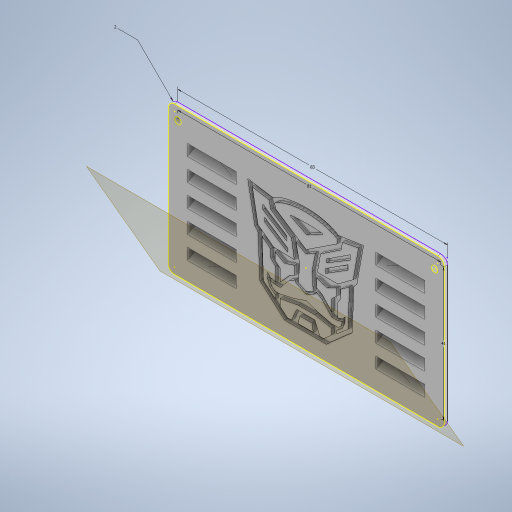
# Autodesk Inventor part: BackDoorV1
Saved by Autodesk Inventor 2024 (Build 280153000, 153)
## iProperties
Created: 2025-05-22
Part Number: BackDoorV1
Material: Ogólny
Document SubType Name: Modeling
Designer: Victoria
Density: 1 g/cm^3
Appearance: Domyślna
Author: Victoria
Autodesk Inventor part; units mm, degrees
ref_plane "YZ Plane" through (0, 0, 0) normal (1, 0, 0) x (0, 1, 0)
ref_plane "XZ Plane" through (0, 0, 0) normal (0, 1, 0) x (-1, 0, 0)
ref_plane "XY Plane" through (0, 0, 0) normal (0, 0, 1) x (1, 0, 0)
sketch "Szkic1" plane through (0, 0, 0) normal (0, 0, 1) x (1, 0, 0)
  line L0 (-40.5, -20.5) -> (40.5, -20.5)
  line L1 (40.5, -20.5) -> (40.5, 20.5)
  line L2 (40.5, 20.5) -> (-40.5, 20.5)
  line L3 (-40.5, 20.5) -> (-40.5, -20.5)
  line L4 (-40.5, -20.5) -> (40.5, 20.5) construction
  line L5 (40.5, -20.5) -> (-40.5, 20.5) construction
  line L6 (-40.5, -22) -> (40.5, -22)
  line L7 (-42.5, 20.5) -> (-42.5, -20)
  line L8 (-40.5, 23.5) -> (40.5, 23.5)
  line L9 (42.5, 21.5) -> (42.5, -20)
  line L10 (40.5, -22) -> (40.5, -22)
  line L11 (-40.5, -22) -> (-40.5, -22)
  line L12 (-42.5, 20.5) -> (-42.5, 21.5)
  line L13 (-40.5, 23.5) -> (-40.5, 23.5)
  arc A0 (-40.5, 23.5) -> (-42.5, 21.5) centre (-40.5, 21.5) ccw
  arc A1 (-42.5, -20) -> (-40.5, -22) centre (-40.5, -20) ccw
  arc A2 (40.5, -22) -> (42.5, -20) centre (40.5, -20) ccw
  arc A3 (42.5, 21.5) -> (40.5, 23.5) centre (40.5, 21.5) ccw
  point P0 (0, 0)
  point P1 (42.5, 23.5)
  point P2 (-42.5, 23.5)
  dimension "d0" = 81
  dimension "d1" = 41
  dimension "d2" = 83
  dimension "d3" = 2
  constraints: 28 end point, 8 point on circle, 8 tangent, 6 point on line, 5 perpendicular, 4 centre point, 3 equal length, 3 equal radius, 3 horizontal, 2 midpoint, 1 vertical
  measures "d0" distance of L2.end L1.end
  measures "d1" distance of L1.end L0.end
  measures "d2" distance of L8.start point (42.5, 23.5)
  measures "d3" radius of A0
extrude "Wyciągnięcie proste1" add sketch "Szkic1" along normal blind 1 contours L3 L2 L1 L0 | A1 L7 L12 A0 L8 A3 L9 A2 L6
extrude "Wyciągnięcie proste2" add sketch "Szkic1" against normal blind 2 contours L3 L2 L1 L0
sketch "Szkic2" plane through (0, 0, -2) normal (0, 0, -1) x (-1, 0, 0)
  circle A0 centre (-39.5, 19.5) radius 1
  line L0 (-40.5, -20.5) -> (-40.5, 20.5) projected
  circle A1 centre (39.5, 19.5) radius 1
  line L1 (40.5, -20.5) -> (40.5, 20.5) projected
  point P0 (0, 0)
  constraints: 2 centre point, 2 tangent
extrude "Wyciągnięcie proste3" cut sketch "Szkic2" against normal through all
sketch "Szkic3" plane through (0, 0, 1) normal (0, 0, 1) x (1, 0, 0)
  circle A0 centre (-39.5, 19.5) radius 1 projected
  circle A1 centre (39.5, 19.5) radius 1 projected
  arc A2 (-42.5, -20) -> (-40.5, -22) centre (-40.5, -20) ccw projected
  line L0 (-40.5, -22) -> (40.5, -22) projected
  arc A3 (40.5, -22) -> (42.5, -20) centre (40.5, -20) ccw projected
  line L1 (42.5, -20) -> (42.5, 21.5) projected
  arc A4 (42.5, 21.5) -> (40.5, 23.5) centre (40.5, 21.5) ccw projected
  line L2 (40.5, 23.5) -> (-40.5, 23.5) projected
  arc A5 (-40.5, 23.5) -> (-42.5, 21.5) centre (-40.5, 21.5) ccw projected
  line L3 (-42.5, 21.5) -> (-42.5, -20) projected
  line L4 (-42.5, 21.5) -> (-42.5, -20) projected
  line L5 (-16.5514, 13.3947) -> (-14.8189, 4.1445)
  line L6 (-14.8189, 4.1445) -> (-9.9927, 0.5868)
  line L7 (-9.9927, 0.5868) -> (-3.6196, 0.3702)
  line L8 (-3.6196, 0.3702) -> (-4.455, 5.7533)
  line L9 (-4.455, 5.7533) -> (-10.8899, 10.1773)
  line L10 (-10.8899, 10.1773) -> (-11.323, 12.4666)
  line L11 (-11.323, 12.4666) -> (-16.5514, 13.3947)
  line L12 (-13.303, 8.9045) -> (-13.303, 10.2966)
  line L13 (-13.303, 10.2966) -> (-5.9709, 5.6561)
  line L14 (-5.9709, 5.6561) -> (-5.9709, 4.233)
  line L15 (-5.9709, 4.233) -> (-13.303, 8.9045)
  line L16 (-12.7461, 5.8726) -> (-12.7461, 7.1101)
  line L17 (-12.7461, 7.1101) -> (-5.7234, 2.5624)
  line L18 (-5.7234, 2.5624) -> (-5.7234, 1.3558)
  line L19 (-5.7234, 1.3558) -> (-12.7461, 5.8726)
  line L20 (4.455, 5.9698) -> (10.7352, 10.1773)
  line L21 (10.7352, 10.1773) -> (11.2302, 12.4666)
  line L22 (11.2302, 12.4666) -> (16.1492, 13.3947)
  line L23 (16.1492, 13.3947) -> (14.5405, 4.1445)
  line L24 (14.5405, 4.1445) -> (9.7761, 0.5868)
  line L25 (9.7761, 0.5868) -> (3.4959, 0.5868)
  line L26 (3.4959, 0.5868) -> (4.455, 5.9698)
  line L27 (6.3421, 4.5114) -> (6.3421, 5.5633)
  line L28 (6.3421, 5.5633) -> (13.5814, 10.2966)
  line L29 (13.5814, 10.2966) -> (13.5814, 8.9045)
  line L30 (13.5814, 8.9045) -> (6.3421, 4.5114)
  line L31 (6.0018, 1.5414) -> (6.0018, 2.8408)
  line L32 (6.0018, 2.8408) -> (12.9008, 7.2957)
  line L33 (12.9008, 7.2957) -> (12.9008, 5.8726)
  line L34 (12.9008, 5.8726) -> (6.0018, 1.5414)
  line L35 (-9.4049, 11.1054) -> (-9.6833, 12.4666)
  line L36 (-9.6833, 12.4666) -> (-9.1144, 12.834)
  line L37 (-9.1144, 12.834) -> (-8.3961, 13.2106)
  line L38 (-8.3961, 13.2106) -> (-7.3824, 13.6422)
  line L39 (-7.3824, 13.6422) -> (-6.0685, 14.0739)
  line L40 (-6.0685, 14.0739) -> (-5.2975, 14.2725)
  line L41 (-5.2975, 14.2725) -> (-4.4496, 14.4505)
  line L42 (-4.4496, 14.4505) -> (-3.5244, 14.6009)
  line L43 (-3.5244, 14.6009) -> (-2.5212, 14.7168)
  line L44 (-2.5212, 14.7168) -> (-1.4394, 14.7914)
  line L45 (-1.4394, 14.7914) -> (-0.2784, 14.8179)
  line L46 (-0.2784, 14.8179) -> (0.8898, 14.7914)
  line L47 (0.8898, 14.7914) -> (1.9922, 14.7168)
  line L48 (1.9922, 14.7168) -> (3.0275, 14.6009)
  line L49 (3.0275, 14.6009) -> (3.9943, 14.4505)
  line L50 (3.9943, 14.4505) -> (4.8913, 14.2725)
  line L51 (4.8913, 14.2725) -> (5.7172, 14.0739)
  line L52 (5.7172, 14.0739) -> (7.1504, 13.6422)
  line L53 (7.1504, 13.6422) -> (8.2834, 13.2106)
  line L54 (8.2834, 13.2106) -> (9.1057, 12.834)
  line L55 (9.1057, 12.834) -> (9.7761, 12.4666)
  line L56 (9.7761, 12.4666) -> (9.4668, 11.1054)
  line L57 (9.4668, 11.1054) -> (0, 4.887)
  line L58 (0, 4.887) -> (-9.4049, 11.1054)
  line L59 (-4.8881, 11.5032) -> (0.2166, 8.9045)
  line L60 (0.2166, 8.9045) -> (5.1356, 11.5032)
  line L61 (5.1356, 11.5032) -> (5.0587, 11.5752)
  line L62 (5.0587, 11.5752) -> (4.8762, 11.6484)
  line L63 (4.8762, 11.6484) -> (4.5207, 11.7313)
  line L64 (4.5207, 11.7313) -> (3.9346, 11.8128)
  line L65 (3.9346, 11.8128) -> (3.0604, 11.8817)
  line L66 (3.0604, 11.8817) -> (1.8402, 11.9266)
  line L67 (1.8402, 11.9266) -> (0.2166, 11.9363)
  line L68 (0.2166, 11.9363) -> (-1.4151, 11.9088)
  line L69 (-1.4151, 11.9088) -> (-2.6562, 11.8556)
  line L70 (-2.6562, 11.8556) -> (-3.5603, 11.7856)
  line L71 (-3.5603, 11.7856) -> (-4.1804, 11.7081)
  line L72 (-4.1804, 11.7081) -> (-4.5699, 11.632)
  line L73 (-4.5699, 11.632) -> (-4.7822, 11.5665)
  line L74 (-4.7822, 11.5665) -> (-4.8881, 11.5032)
  line L75 (-3.0937, 5.3511) -> (0, 3.7114)
  line L76 (0, 3.7114) -> (2.8772, 5.3511)
  line L77 (2.8772, 5.3511) -> (1.8253, -0.0629)
  line L78 (1.8253, -0.0629) -> (2.2275, -5.1675)
  line L79 (2.2275, -5.1675) -> (0, -6.3432)
  line L80 (0, -6.3432) -> (-2.444, -5.1675)
  line L81 (-2.444, -5.1675) -> (-1.949, -0.0629)
  line L82 (-1.949, -0.0629) -> (-3.0937, 5.3511)
  line L83 (-7.9818, -7.7972) -> (-5.1046, -4.5488)
  line L84 (-5.1046, -4.5488) -> (-3.434, -3.6516)
  line L85 (-3.434, -3.6516) -> (-3.434, -1.022)
  line L86 (-3.434, -1.022) -> (-6.6206, -2.0738)
  line L87 (-6.6206, -2.0738) -> (-9.5596, -0.4651)
  line L88 (-9.5596, -0.4651) -> (-9.5596, -2.7854)
  line L89 (-9.5596, -2.7854) -> (-7.9818, -4.0538)
  line L90 (-7.9818, -4.0538) -> (-7.9818, -7.7972)
  line L91 (-13.5195, 1.6386) -> (-13.1483, -9.9009)
  line L92 (-13.1483, -9.9009) -> (-9.4049, -13.0565)
  line L93 (-9.4049, -13.0565) -> (-9.4049, -11.9118)
  line L94 (-9.4049, -11.9118) -> (-11.1374, -10.5197)
  line L95 (-11.1374, -10.5197) -> (-11.8489, -8.6944)
  line L96 (-11.8489, -8.6944) -> (-11.8489, -7.0857)
  line L97 (-11.8489, -7.0857) -> (-11.1374, -7.9828)
  line L98 (-11.1374, -7.9828) -> (-9.4049, -8.4778)
  line L99 (-9.4049, -8.4778) -> (-9.4049, -4.3013)
  line L100 (-9.4049, -4.3013) -> (-10.8899, -2.7854)
  line L101 (-10.8899, -2.7854) -> (-10.8899, -0.3104)
  line L102 (-10.8899, -0.3104) -> (-13.5195, 1.6386)
  line L103 (-3.434, -4.92) -> (-3.0937, -5.5035)
  line L104 (-3.0937, -5.5035) -> (-2.444, -5.7819)
  line L105 (-2.444, -5.7819) -> (0, -7.0194)
  line L106 (0, -7.0194) -> (2.3512, -5.7819)
  line L107 (2.3512, -5.7819) -> (2.8772, -5.5035)
  line L108 (2.8772, -5.5035) -> (3.2175, -4.92)
  line L109 (3.2175, -4.92) -> (4.919, -5.91)
  line L110 (4.919, -5.91) -> (7.889, -9.1584)
  line L111 (7.889, -9.1584) -> (9.7761, -9.1584)
  line L112 (9.7761, -9.1584) -> (11.2302, -8.6944)
  line L113 (11.2302, -8.6944) -> (10.7352, -10.2412)
  line L114 (10.7352, -10.2412) -> (9.7761, -10.9528)
  line L115 (9.7761, -10.9528) -> (7.889, -10.9528)
  line L116 (7.889, -10.9528) -> (3.4959, -9.9009)
  line L117 (3.4959, -9.9009) -> (0, -8.6944)
  line L118 (0, -8.6944) -> (-3.434, -9.9009)
  line L119 (-3.434, -9.9009) -> (-7.9818, -10.9528)
  line L120 (-7.9818, -10.9528) -> (-9.6833, -10.9528)
  line L121 (-9.6833, -10.9528) -> (-10.7043, -10.0512)
  line L122 (-10.7043, -10.0512) -> (-11.1374, -8.6944)
  line L123 (-11.1374, -8.6944) -> (-9.6833, -9.1584)
  line L124 (-9.6833, -9.1584) -> (-7.9818, -9.1584)
  line L125 (-7.9818, -9.1584) -> (-5.1046, -5.91)
  line L126 (-5.1046, -5.91) -> (-3.434, -4.92)
  line L127 (7.889, -13.9537) -> (5.414, -16.1502)
  line L128 (5.414, -16.1502) -> (4.2075, -16.1502)
  line L129 (4.2075, -16.1502) -> (2.6915, -12.4997)
  line L130 (2.6915, -12.4997) -> (-2.8772, -12.4997)
  line L131 (-2.8772, -12.4997) -> (-4.455, -16.1502)
  line L132 (-4.455, -16.1502) -> (-5.7234, -16.1502)
  line L133 (-5.7234, -16.1502) -> (-7.9818, -14.2631)
  line L134 (-7.9818, -14.2631) -> (-7.9818, -12.1284)
  line L135 (-7.9818, -12.1284) -> (-2.444, -11.1384)
  line L136 (-2.444, -11.1384) -> (2.6915, -11.1384)
  line L137 (2.6915, -11.1384) -> (7.889, -12.1284)
  line L138 (7.889, -12.1284) -> (7.889, -13.9537)
  line L139 (-2.444, -16.0574) -> (2.2275, -16.0574)
  line L140 (2.2275, -16.0574) -> (1.8253, -13.7681)
  line L141 (1.8253, -13.7681) -> (-1.949, -13.7681)
  line L142 (-1.949, -13.7681) -> (-2.444, -16.0574)
  line L143 (3.2175, -1.022) -> (3.2175, -3.6516)
  line L144 (3.2175, -3.6516) -> (4.919, -4.5488)
  line L145 (4.919, -4.5488) -> (7.889, -7.7972)
  line L146 (7.889, -7.7972) -> (7.889, -4.3013)
  line L147 (7.889, -4.3013) -> (9.4668, -2.7854)
  line L148 (9.4668, -2.7854) -> (9.4668, -0.6198)
  line L149 (9.4668, -0.6198) -> (6.5277, -2.0738)
  line L150 (6.5277, -2.0738) -> (3.2175, -1.022)
  line L151 (10.7352, -0.3104) -> (13.3649, 1.6386)
  line L152 (13.3649, 1.6386) -> (12.9317, -9.9009)
  line L153 (12.9317, -9.9009) -> (9.4668, -12.84)
  line L154 (9.4668, -12.84) -> (9.4668, -11.9118)
  line L155 (9.4668, -11.9118) -> (11.2302, -10.5197)
  line L156 (11.2302, -10.5197) -> (11.9727, -8.6944)
  line L157 (11.9727, -8.6944) -> (11.9727, -7.0857)
  line L158 (11.9727, -7.0857) -> (11.2302, -7.9828)
  line L159 (11.2302, -7.9828) -> (9.7761, -8.4778)
  line L160 (9.7761, -8.4778) -> (9.7761, -4.3013)
  line L161 (9.7761, -4.3013) -> (10.7352, -2.7854)
  line L162 (10.7352, -2.7854) -> (10.7352, -0.3104)
  line L163 (-6.6206, -17.2021) -> (-14.2002, -10.5197)
  line L164 (-14.2002, -10.5197) -> (-14.8189, 2.4739)
  line L165 (-14.8189, 2.4739) -> (-15.747, 3.3711)
  line L166 (-15.747, 3.3711) -> (-17.9436, 14.8179)
  line L167 (-17.9436, 14.8179) -> (-10.3021, 13.6732)
  line L168 (-10.3021, 13.6732) -> (-9.693, 14.0328)
  line L169 (-9.693, 14.0328) -> (-8.9251, 14.4041)
  line L170 (-8.9251, 14.4041) -> (-7.8426, 14.8333)
  line L171 (-7.8426, 14.8333) -> (-6.441, 15.2684)
  line L172 (-6.441, 15.2684) -> (-5.6192, 15.4718)
  line L173 (-5.6192, 15.4718) -> (-4.716, 15.657)
  line L174 (-4.716, 15.657) -> (-3.7309, 15.8176)
  line L175 (-3.7309, 15.8176) -> (-2.6633, 15.9471)
  line L176 (-2.6633, 15.9471) -> (-1.5126, 16.0388)
  line L177 (-1.5126, 16.0388) -> (-0.2784, 16.0863)
  line L178 (-0.2784, 16.0863) -> (0.9589, 16.0796)
  line L179 (0.9589, 16.0796) -> (2.1183, 16.0181)
  line L180 (2.1183, 16.0181) -> (3.1997, 15.9095)
  line L181 (3.1997, 15.9095) -> (4.2026, 15.7614)
  line L182 (4.2026, 15.7614) -> (5.1269, 15.5814)
  line L183 (5.1269, 15.5814) -> (5.9722, 15.3771)
  line L184 (5.9722, 15.3771) -> (7.4249, 14.9261)
  line L185 (7.4249, 14.9261) -> (8.5586, 14.4693)
  line L186 (8.5586, 14.4693) -> (9.3711, 14.0676)
  line L187 (9.3711, 14.0676) -> (10.0236, 13.6732)
  line L188 (10.0236, 13.6732) -> (17.6961, 14.8179)
  line L189 (17.6961, 14.8179) -> (15.6233, 3.3711)
  line L190 (15.6233, 3.3711) -> (14.757, 2.4739)
  line L191 (14.757, 2.4739) -> (14.1692, -10.2412)
  line L192 (14.1692, -10.2412) -> (6.2802, -17.2021)
  line L193 (6.2802, -17.2021) -> (-6.6206, -17.2021)
  line L194 (-14.8189, 4.1445) -> (-16.5514, 13.3947)
  line L195 (-16.5514, 13.3947) -> (-11.323, 12.4666)
  line L196 (-11.323, 12.4666) -> (-10.8899, 10.1773)
  line L197 (-10.8899, 10.1773) -> (-4.455, 5.7533)
  line L198 (-4.455, 5.7533) -> (-3.6196, 0.3702)
  line L199 (-3.6196, 0.3702) -> (-9.9927, 0.5868)
  line L200 (-9.9927, 0.5868) -> (-14.8189, 4.1445)
  line L201 (-9.6833, 12.4666) -> (-9.4049, 11.1054)
  line L202 (-9.4049, 11.1054) -> (0, 4.887)
  line L203 (0, 4.887) -> (9.4668, 11.1054)
  line L204 (9.4668, 11.1054) -> (9.7761, 12.4666)
  line L205 (9.7761, 12.4666) -> (9.1057, 12.834)
  line L206 (9.1057, 12.834) -> (8.2834, 13.2106)
  line L207 (8.2834, 13.2106) -> (7.1504, 13.6422)
  line L208 (7.1504, 13.6422) -> (5.7172, 14.0739)
  line L209 (5.7172, 14.0739) -> (4.8913, 14.2725)
  line L210 (4.8913, 14.2725) -> (3.9943, 14.4505)
  line L211 (3.9943, 14.4505) -> (3.0275, 14.6009)
  line L212 (3.0275, 14.6009) -> (1.9922, 14.7168)
  line L213 (1.9922, 14.7168) -> (0.8898, 14.7914)
  line L214 (0.8898, 14.7914) -> (-0.2784, 14.8179)
  line L215 (-0.2784, 14.8179) -> (-1.4394, 14.7914)
  line L216 (-1.4394, 14.7914) -> (-2.5212, 14.7168)
  line L217 (-2.5212, 14.7168) -> (-3.5244, 14.6009)
  line L218 (-3.5244, 14.6009) -> (-4.4496, 14.4505)
  line L219 (-4.4496, 14.4505) -> (-5.2975, 14.2725)
  line L220 (-5.2975, 14.2725) -> (-6.0685, 14.0739)
  line L221 (-6.0685, 14.0739) -> (-7.3824, 13.6422)
  line L222 (-7.3824, 13.6422) -> (-8.3961, 13.2106)
  line L223 (-8.3961, 13.2106) -> (-9.1144, 12.834)
  line L224 (-9.1144, 12.834) -> (-9.6833, 12.4666)
  line L225 (0, 3.7114) -> (-3.0937, 5.3511)
  line L226 (-3.0937, 5.3511) -> (-1.949, -0.0629)
  line L227 (-1.949, -0.0629) -> (-2.444, -5.1675)
  line L228 (-2.444, -5.1675) -> (0, -6.3432)
  line L229 (0, -6.3432) -> (2.2275, -5.1675)
  line L230 (2.2275, -5.1675) -> (1.8253, -0.0629)
  line L231 (1.8253, -0.0629) -> (2.8772, 5.3511)
  line L232 (2.8772, 5.3511) -> (0, 3.7114)
  line L233 (10.7352, 10.1773) -> (4.455, 5.9698)
  line L234 (4.455, 5.9698) -> (3.4959, 0.5868)
  line L235 (3.4959, 0.5868) -> (9.7761, 0.5868)
  line L236 (9.7761, 0.5868) -> (14.5405, 4.1445)
  line L237 (14.5405, 4.1445) -> (16.1492, 13.3947)
  line L238 (16.1492, 13.3947) -> (11.2302, 12.4666)
  line L239 (11.2302, 12.4666) -> (10.7352, 10.1773)
  line L240 (-2.444, -5.7819) -> (-3.0937, -5.5035)
  line L241 (-3.0937, -5.5035) -> (-3.434, -4.92)
  line L242 (-3.434, -4.92) -> (-5.1046, -5.91)
  line L243 (-5.1046, -5.91) -> (-7.9818, -9.1584)
  line L244 (-7.9818, -9.1584) -> (-9.6833, -9.1584)
  line L245 (-9.6833, -9.1584) -> (-11.1374, -8.6944)
  line L246 (-11.1374, -8.6944) -> (-10.7043, -10.0512)
  line L247 (-10.7043, -10.0512) -> (-9.6833, -10.9528)
  line L248 (-9.6833, -10.9528) -> (-7.9818, -10.9528)
  line L249 (-7.9818, -10.9528) -> (-3.434, -9.9009)
  line L250 (-3.434, -9.9009) -> (0, -8.6944)
  line L251 (0, -8.6944) -> (3.4959, -9.9009)
  line L252 (3.4959, -9.9009) -> (7.889, -10.9528)
  line L253 (7.889, -10.9528) -> (9.7761, -10.9528)
  line L254 (9.7761, -10.9528) -> (10.7352, -10.2412)
  line L255 (10.7352, -10.2412) -> (11.2302, -8.6944)
  line L256 (11.2302, -8.6944) -> (9.7761, -9.1584)
  line L257 (9.7761, -9.1584) -> (7.889, -9.1584)
  line L258 (7.889, -9.1584) -> (4.919, -5.91)
  line L259 (4.919, -5.91) -> (3.2175, -4.92)
  line L260 (3.2175, -4.92) -> (2.8772, -5.5035)
  line L261 (2.8772, -5.5035) -> (2.3512, -5.7819)
  line L262 (2.3512, -5.7819) -> (0, -7.0194)
  line L263 (0, -7.0194) -> (-2.444, -5.7819)
  line L264 (-13.1483, -9.9009) -> (-13.5195, 1.6386)
  line L265 (-13.5195, 1.6386) -> (-10.8899, -0.3104)
  line L266 (-10.8899, -0.3104) -> (-10.8899, -2.7854)
  line L267 (-10.8899, -2.7854) -> (-9.4049, -4.3013)
  line L268 (-9.4049, -4.3013) -> (-9.4049, -8.4778)
  line L269 (-9.4049, -8.4778) -> (-11.1374, -7.9828)
  line L270 (-11.1374, -7.9828) -> (-11.8489, -7.0857)
  line L271 (-11.8489, -7.0857) -> (-11.8489, -8.6944)
  line L272 (-11.8489, -8.6944) -> (-11.1374, -10.5197)
  line L273 (-11.1374, -10.5197) -> (-9.4049, -11.9118)
  line L274 (-9.4049, -11.9118) -> (-9.4049, -13.0565)
  line L275 (-9.4049, -13.0565) -> (-13.1483, -9.9009)
  line L276 (2.2275, -16.0574) -> (-2.444, -16.0574)
  line L277 (-2.444, -16.0574) -> (-1.949, -13.7681)
  line L278 (-1.949, -13.7681) -> (1.8253, -13.7681)
  line L279 (1.8253, -13.7681) -> (2.2275, -16.0574)
  line L280 (3.2175, -3.6516) -> (3.2175, -1.022)
  line L281 (3.2175, -1.022) -> (6.5277, -2.0738)
  line L282 (6.5277, -2.0738) -> (9.4668, -0.6198)
  line L283 (9.4668, -0.6198) -> (9.4668, -2.7854)
  line L284 (9.4668, -2.7854) -> (7.889, -4.3013)
  line L285 (7.889, -4.3013) -> (7.889, -7.7972)
  line L286 (7.889, -7.7972) -> (4.919, -4.5488)
  line L287 (4.919, -4.5488) -> (3.2175, -3.6516)
  line L288 (13.3649, 1.6386) -> (10.7352, -0.3104)
  line L289 (10.7352, -0.3104) -> (10.7352, -2.7854)
  line L290 (10.7352, -2.7854) -> (9.7761, -4.3013)
  line L291 (9.7761, -4.3013) -> (9.7761, -8.4778)
  line L292 (9.7761, -8.4778) -> (11.2302, -7.9828)
  line L293 (11.2302, -7.9828) -> (11.9727, -7.0857)
  line L294 (11.9727, -7.0857) -> (11.9727, -8.6944)
  line L295 (11.9727, -8.6944) -> (11.2302, -10.5197)
  line L296 (11.2302, -10.5197) -> (9.4668, -11.9118)
  line L297 (9.4668, -11.9118) -> (9.4668, -12.84)
  line L298 (9.4668, -12.84) -> (12.9317, -9.9009)
  line L299 (12.9317, -9.9009) -> (13.3649, 1.6386)
  line L300 (5.414, -16.1502) -> (7.889, -13.9537)
  line L301 (7.889, -13.9537) -> (7.889, -12.1284)
  line L302 (7.889, -12.1284) -> (2.6915, -11.1384)
  line L303 (2.6915, -11.1384) -> (-2.444, -11.1384)
  line L304 (-2.444, -11.1384) -> (-7.9818, -12.1284)
  line L305 (-7.9818, -12.1284) -> (-7.9818, -14.2631)
  line L306 (-7.9818, -14.2631) -> (-5.7234, -16.1502)
  line L307 (-5.7234, -16.1502) -> (-4.455, -16.1502)
  line L308 (-4.455, -16.1502) -> (-2.8772, -12.4997)
  line L309 (-2.8772, -12.4997) -> (2.6915, -12.4997)
  line L310 (2.6915, -12.4997) -> (4.2075, -16.1502)
  line L311 (4.2075, -16.1502) -> (5.414, -16.1502)
  line L312 (-5.1046, -4.5488) -> (-7.9818, -7.7972)
  line L313 (-7.9818, -7.7972) -> (-7.9818, -4.0538)
  line L314 (-7.9818, -4.0538) -> (-9.5596, -2.7854)
  line L315 (-9.5596, -2.7854) -> (-9.5596, -0.4651)
  line L316 (-9.5596, -0.4651) -> (-6.6206, -2.0738)
  line L317 (-6.6206, -2.0738) -> (-3.434, -1.022)
  line L318 (-3.434, -1.022) -> (-3.434, -3.6516)
  line L319 (-3.434, -3.6516) -> (-5.1046, -4.5488)
  line L320 (6.0018, 2.8408) -> (6.0018, 1.5414)
  line L321 (6.0018, 1.5414) -> (12.9008, 5.8726)
  line L322 (12.9008, 5.8726) -> (12.9008, 7.2957)
  line L323 (12.9008, 7.2957) -> (6.0018, 2.8408)
  line L324 (6.3421, 5.5633) -> (6.3421, 4.5114)
  line L325 (6.3421, 4.5114) -> (13.5814, 8.9045)
  line L326 (13.5814, 8.9045) -> (13.5814, 10.2966)
  line L327 (13.5814, 10.2966) -> (6.3421, 5.5633)
  line L328 (0.2166, 8.9045) -> (-4.8881, 11.5032)
  line L329 (-4.8881, 11.5032) -> (-4.7822, 11.5665)
  line L330 (-4.7822, 11.5665) -> (-4.5699, 11.632)
  line L331 (-4.5699, 11.632) -> (-4.1804, 11.7081)
  line L332 (-4.1804, 11.7081) -> (-3.5603, 11.7856)
  line L333 (-3.5603, 11.7856) -> (-2.6562, 11.8556)
  line L334 (-2.6562, 11.8556) -> (-1.4151, 11.9088)
  line L335 (-1.4151, 11.9088) -> (0.2166, 11.9363)
  line L336 (0.2166, 11.9363) -> (1.8402, 11.9266)
  line L337 (1.8402, 11.9266) -> (3.0604, 11.8817)
  line L338 (3.0604, 11.8817) -> (3.9346, 11.8128)
  line L339 (3.9346, 11.8128) -> (4.5207, 11.7313)
  line L340 (4.5207, 11.7313) -> (4.8762, 11.6484)
  line L341 (4.8762, 11.6484) -> (5.0587, 11.5752)
  line L342 (5.0587, 11.5752) -> (5.1356, 11.5032)
  line L343 (5.1356, 11.5032) -> (0.2166, 8.9045)
  line L344 (-13.303, 10.2966) -> (-13.303, 8.9045)
  line L345 (-13.303, 8.9045) -> (-5.9709, 4.233)
  line L346 (-5.9709, 4.233) -> (-5.9709, 5.6561)
  line L347 (-5.9709, 5.6561) -> (-13.303, 10.2966)
  line L348 (-12.7461, 7.1101) -> (-12.7461, 5.8726)
  line L349 (-12.7461, 5.8726) -> (-5.7234, 1.3558)
  line L350 (-5.7234, 1.3558) -> (-5.7234, 2.5624)
  line L351 (-5.7234, 2.5624) -> (-12.7461, 7.1101)
  line L352 (-16.5514, 13.3947) -> (-14.8189, 4.1445)
  line L353 (-14.8189, 4.1445) -> (-9.9927, 0.5868)
  line L354 (-9.9927, 0.5868) -> (-3.6196, 0.3702)
  line L355 (-3.6196, 0.3702) -> (-4.455, 5.7533)
  line L356 (-4.455, 5.7533) -> (-10.8899, 10.1773)
  line L357 (-10.8899, 10.1773) -> (-11.323, 12.4666)
  line L358 (-11.323, 12.4666) -> (-16.5514, 13.3947)
  line L359 (-13.303, 8.9045) -> (-13.303, 10.2966)
  line L360 (-13.303, 10.2966) -> (-5.9709, 5.6561)
  line L361 (-5.9709, 5.6561) -> (-5.9709, 4.233)
  line L362 (-5.9709, 4.233) -> (-13.303, 8.9045)
  line L363 (-12.7461, 5.8726) -> (-12.7461, 7.1101)
  line L364 (-12.7461, 7.1101) -> (-5.7234, 2.5624)
  line L365 (-5.7234, 2.5624) -> (-5.7234, 1.3558)
  line L366 (-5.7234, 1.3558) -> (-12.7461, 5.8726)
  line L367 (4.455, 5.9698) -> (10.7352, 10.1773)
  line L368 (10.7352, 10.1773) -> (11.2302, 12.4666)
  line L369 (11.2302, 12.4666) -> (16.1492, 13.3947)
  line L370 (16.1492, 13.3947) -> (14.5405, 4.1445)
  line L371 (14.5405, 4.1445) -> (9.7761, 0.5868)
  line L372 (9.7761, 0.5868) -> (3.4959, 0.5868)
  line L373 (3.4959, 0.5868) -> (4.455, 5.9698)
  line L374 (6.3421, 4.5114) -> (6.3421, 5.5633)
  line L375 (6.3421, 5.5633) -> (13.5814, 10.2966)
  line L376 (13.5814, 10.2966) -> (13.5814, 8.9045)
  line L377 (13.5814, 8.9045) -> (6.3421, 4.5114)
  line L378 (6.0018, 1.5414) -> (6.0018, 2.8408)
  line L379 (6.0018, 2.8408) -> (12.9008, 7.2957)
  line L380 (12.9008, 7.2957) -> (12.9008, 5.8726)
  line L381 (12.9008, 5.8726) -> (6.0018, 1.5414)
  line L382 (-9.4049, 11.1054) -> (-9.6833, 12.4666)
  line L383 (-9.6833, 12.4666) -> (-9.1144, 12.834)
  line L384 (-9.1144, 12.834) -> (-8.3961, 13.2106)
  line L385 (-8.3961, 13.2106) -> (-7.3824, 13.6422)
  line L386 (-7.3824, 13.6422) -> (-6.0685, 14.0739)
  line L387 (-6.0685, 14.0739) -> (-5.2975, 14.2725)
  line L388 (-5.2975, 14.2725) -> (-4.4496, 14.4505)
  line L389 (-4.4496, 14.4505) -> (-3.5244, 14.6009)
  line L390 (-3.5244, 14.6009) -> (-2.5212, 14.7168)
  line L391 (-2.5212, 14.7168) -> (-1.4394, 14.7914)
  line L392 (-1.4394, 14.7914) -> (-0.2784, 14.8179)
  line L393 (-0.2784, 14.8179) -> (0.8898, 14.7914)
  line L394 (0.8898, 14.7914) -> (1.9922, 14.7168)
  line L395 (1.9922, 14.7168) -> (3.0275, 14.6009)
  line L396 (3.0275, 14.6009) -> (3.9943, 14.4505)
  line L397 (3.9943, 14.4505) -> (4.8913, 14.2725)
  line L398 (4.8913, 14.2725) -> (5.7172, 14.0739)
  line L399 (5.7172, 14.0739) -> (7.1504, 13.6422)
  line L400 (7.1504, 13.6422) -> (8.2834, 13.2106)
  line L401 (8.2834, 13.2106) -> (9.1057, 12.834)
  line L402 (9.1057, 12.834) -> (9.7761, 12.4666)
  line L403 (9.7761, 12.4666) -> (9.4668, 11.1054)
  line L404 (9.4668, 11.1054) -> (0, 4.887)
  line L405 (0, 4.887) -> (-9.4049, 11.1054)
  line L406 (-4.8881, 11.5032) -> (0.2166, 8.9045)
  line L407 (0.2166, 8.9045) -> (5.1356, 11.5032)
  line L408 (5.1356, 11.5032) -> (5.0587, 11.5752)
  line L409 (5.0587, 11.5752) -> (4.8762, 11.6484)
  line L410 (4.8762, 11.6484) -> (4.5207, 11.7313)
  line L411 (4.5207, 11.7313) -> (3.9346, 11.8128)
  line L412 (3.9346, 11.8128) -> (3.0604, 11.8817)
  line L413 (3.0604, 11.8817) -> (1.8402, 11.9266)
  line L414 (1.8402, 11.9266) -> (0.2166, 11.9363)
  line L415 (0.2166, 11.9363) -> (-1.4151, 11.9088)
  line L416 (-1.4151, 11.9088) -> (-2.6562, 11.8556)
  line L417 (-2.6562, 11.8556) -> (-3.5603, 11.7856)
  line L418 (-3.5603, 11.7856) -> (-4.1804, 11.7081)
  line L419 (-4.1804, 11.7081) -> (-4.5699, 11.632)
  line L420 (-4.5699, 11.632) -> (-4.7822, 11.5665)
  line L421 (-4.7822, 11.5665) -> (-4.8881, 11.5032)
  line L422 (-3.0937, 5.3511) -> (0, 3.7114)
  line L423 (0, 3.7114) -> (2.8772, 5.3511)
  line L424 (2.8772, 5.3511) -> (1.8253, -0.0629)
  line L425 (1.8253, -0.0629) -> (2.2275, -5.1675)
  line L426 (2.2275, -5.1675) -> (0, -6.3432)
  line L427 (0, -6.3432) -> (-2.444, -5.1675)
  line L428 (-2.444, -5.1675) -> (-1.949, -0.0629)
  line L429 (-1.949, -0.0629) -> (-3.0937, 5.3511)
  line L430 (-7.9818, -7.7972) -> (-5.1046, -4.5488)
  line L431 (-5.1046, -4.5488) -> (-3.434, -3.6516)
  line L432 (-3.434, -3.6516) -> (-3.434, -1.022)
  line L433 (-3.434, -1.022) -> (-6.6206, -2.0738)
  line L434 (-6.6206, -2.0738) -> (-9.5596, -0.4651)
  line L435 (-9.5596, -0.4651) -> (-9.5596, -2.7854)
  line L436 (-9.5596, -2.7854) -> (-7.9818, -4.0538)
  line L437 (-7.9818, -4.0538) -> (-7.9818, -7.7972)
  line L438 (-13.5195, 1.6386) -> (-13.1483, -9.9009)
  line L439 (-13.1483, -9.9009) -> (-9.4049, -13.0565)
  line L440 (-9.4049, -13.0565) -> (-9.4049, -11.9118)
  line L441 (-9.4049, -11.9118) -> (-11.1374, -10.5197)
  line L442 (-11.1374, -10.5197) -> (-11.8489, -8.6944)
  line L443 (-11.8489, -8.6944) -> (-11.8489, -7.0857)
  line L444 (-11.8489, -7.0857) -> (-11.1374, -7.9828)
  line L445 (-11.1374, -7.9828) -> (-9.4049, -8.4778)
  line L446 (-9.4049, -8.4778) -> (-9.4049, -4.3013)
  line L447 (-9.4049, -4.3013) -> (-10.8899, -2.7854)
  line L448 (-10.8899, -2.7854) -> (-10.8899, -0.3104)
  line L449 (-10.8899, -0.3104) -> (-13.5195, 1.6386)
  line L450 (-3.434, -4.92) -> (-3.0937, -5.5035)
  line L451 (-3.0937, -5.5035) -> (-2.444, -5.7819)
  line L452 (-2.444, -5.7819) -> (0, -7.0194)
  line L453 (0, -7.0194) -> (2.3512, -5.7819)
  line L454 (2.3512, -5.7819) -> (2.8772, -5.5035)
  line L455 (2.8772, -5.5035) -> (3.2175, -4.92)
  line L456 (3.2175, -4.92) -> (4.919, -5.91)
  line L457 (4.919, -5.91) -> (7.889, -9.1584)
  line L458 (7.889, -9.1584) -> (9.7761, -9.1584)
  line L459 (9.7761, -9.1584) -> (11.2302, -8.6944)
  line L460 (11.2302, -8.6944) -> (10.7352, -10.2412)
  line L461 (10.7352, -10.2412) -> (9.7761, -10.9528)
  line L462 (9.7761, -10.9528) -> (7.889, -10.9528)
  line L463 (7.889, -10.9528) -> (3.4959, -9.9009)
  line L464 (3.4959, -9.9009) -> (0, -8.6944)
  line L465 (0, -8.6944) -> (-3.434, -9.9009)
  line L466 (-3.434, -9.9009) -> (-7.9818, -10.9528)
  line L467 (-7.9818, -10.9528) -> (-9.6833, -10.9528)
  line L468 (-9.6833, -10.9528) -> (-10.7043, -10.0512)
  line L469 (-10.7043, -10.0512) -> (-11.1374, -8.6944)
  line L470 (-11.1374, -8.6944) -> (-9.6833, -9.1584)
  line L471 (-9.6833, -9.1584) -> (-7.9818, -9.1584)
  line L472 (-7.9818, -9.1584) -> (-5.1046, -5.91)
  line L473 (-5.1046, -5.91) -> (-3.434, -4.92)
  line L474 (7.889, -13.9537) -> (5.414, -16.1502)
  line L475 (5.414, -16.1502) -> (4.2075, -16.1502)
  line L476 (4.2075, -16.1502) -> (2.6915, -12.4997)
  line L477 (2.6915, -12.4997) -> (-2.8772, -12.4997)
  line L478 (-2.8772, -12.4997) -> (-4.455, -16.1502)
  line L479 (-4.455, -16.1502) -> (-5.7234, -16.1502)
  line L480 (-5.7234, -16.1502) -> (-7.9818, -14.2631)
  line L481 (-7.9818, -14.2631) -> (-7.9818, -12.1284)
  line L482 (-7.9818, -12.1284) -> (-2.444, -11.1384)
  line L483 (-2.444, -11.1384) -> (2.6915, -11.1384)
  line L484 (2.6915, -11.1384) -> (7.889, -12.1284)
  line L485 (7.889, -12.1284) -> (7.889, -13.9537)
  line L486 (-2.444, -16.0574) -> (2.2275, -16.0574)
  line L487 (2.2275, -16.0574) -> (1.8253, -13.7681)
  line L488 (1.8253, -13.7681) -> (-1.949, -13.7681)
  line L489 (-1.949, -13.7681) -> (-2.444, -16.0574)
  line L490 (3.2175, -1.022) -> (3.2175, -3.6516)
  line L491 (3.2175, -3.6516) -> (4.919, -4.5488)
  line L492 (4.919, -4.5488) -> (7.889, -7.7972)
  line L493 (7.889, -7.7972) -> (7.889, -4.3013)
  line L494 (7.889, -4.3013) -> (9.4668, -2.7854)
  line L495 (9.4668, -2.7854) -> (9.4668, -0.6198)
  line L496 (9.4668, -0.6198) -> (6.5277, -2.0738)
  line L497 (6.5277, -2.0738) -> (3.2175, -1.022)
  line L498 (10.7352, -0.3104) -> (13.3649, 1.6386)
  line L499 (13.3649, 1.6386) -> (12.9317, -9.9009)
  line L500 (12.9317, -9.9009) -> (9.4668, -12.84)
  line L501 (9.4668, -12.84) -> (9.4668, -11.9118)
  line L502 (9.4668, -11.9118) -> (11.2302, -10.5197)
  line L503 (11.2302, -10.5197) -> (11.9727, -8.6944)
  line L504 (11.9727, -8.6944) -> (11.9727, -7.0857)
  line L505 (11.9727, -7.0857) -> (11.2302, -7.9828)
  line L506 (11.2302, -7.9828) -> (9.7761, -8.4778)
  line L507 (9.7761, -8.4778) -> (9.7761, -4.3013)
  line L508 (9.7761, -4.3013) -> (10.7352, -2.7854)
  line L509 (10.7352, -2.7854) -> (10.7352, -0.3104)
  line L510 (-6.6206, -17.2021) -> (-14.2002, -10.5197)
  line L511 (-14.2002, -10.5197) -> (-14.8189, 2.4739)
  line L512 (-14.8189, 2.4739) -> (-15.747, 3.3711)
  line L513 (-15.747, 3.3711) -> (-17.9436, 14.8179)
  line L514 (-17.9436, 14.8179) -> (-10.3021, 13.6732)
  line L515 (-10.3021, 13.6732) -> (-9.693, 14.0328)
  line L516 (-9.693, 14.0328) -> (-8.9251, 14.4041)
  line L517 (-8.9251, 14.4041) -> (-7.8426, 14.8333)
  line L518 (-7.8426, 14.8333) -> (-6.441, 15.2684)
  line L519 (-6.441, 15.2684) -> (-5.6192, 15.4718)
  line L520 (-5.6192, 15.4718) -> (-4.716, 15.657)
  line L521 (-4.716, 15.657) -> (-3.7309, 15.8176)
  line L522 (-3.7309, 15.8176) -> (-2.6633, 15.9471)
  line L523 (-2.6633, 15.9471) -> (-1.5126, 16.0388)
  line L524 (-1.5126, 16.0388) -> (-0.2784, 16.0863)
  line L525 (-0.2784, 16.0863) -> (0.9589, 16.0796)
  line L526 (0.9589, 16.0796) -> (2.1183, 16.0181)
  line L527 (2.1183, 16.0181) -> (3.1997, 15.9095)
  line L528 (3.1997, 15.9095) -> (4.2026, 15.7614)
  line L529 (4.2026, 15.7614) -> (5.1269, 15.5814)
  line L530 (5.1269, 15.5814) -> (5.9722, 15.3771)
  line L531 (5.9722, 15.3771) -> (7.4249, 14.9261)
  line L532 (7.4249, 14.9261) -> (8.5586, 14.4693)
  line L533 (8.5586, 14.4693) -> (9.3711, 14.0676)
  line L534 (9.3711, 14.0676) -> (10.0236, 13.6732)
  line L535 (10.0236, 13.6732) -> (17.6961, 14.8179)
  line L536 (17.6961, 14.8179) -> (15.6233, 3.3711)
  line L537 (15.6233, 3.3711) -> (14.757, 2.4739)
  line L538 (14.757, 2.4739) -> (14.1692, -10.2412)
  line L539 (14.1692, -10.2412) -> (6.2802, -17.2021)
  line L540 (6.2802, -17.2021) -> (-6.6206, -17.2021)
  line L541 (-14.8189, 4.1445) -> (-16.5514, 13.3947)
  line L542 (-16.5514, 13.3947) -> (-11.323, 12.4666)
  line L543 (-11.323, 12.4666) -> (-10.8899, 10.1773)
  line L544 (-10.8899, 10.1773) -> (-4.455, 5.7533)
  line L545 (-4.455, 5.7533) -> (-3.6196, 0.3702)
  line L546 (-3.6196, 0.3702) -> (-9.9927, 0.5868)
  line L547 (-9.9927, 0.5868) -> (-14.8189, 4.1445)
  line L548 (-9.6833, 12.4666) -> (-9.4049, 11.1054)
  line L549 (-9.4049, 11.1054) -> (0, 4.887)
  line L550 (0, 4.887) -> (9.4668, 11.1054)
  line L551 (9.4668, 11.1054) -> (9.7761, 12.4666)
  line L552 (9.7761, 12.4666) -> (9.1057, 12.834)
  line L553 (9.1057, 12.834) -> (8.2834, 13.2106)
  line L554 (8.2834, 13.2106) -> (7.1504, 13.6422)
  line L555 (7.1504, 13.6422) -> (5.7172, 14.0739)
  line L556 (5.7172, 14.0739) -> (4.8913, 14.2725)
  line L557 (4.8913, 14.2725) -> (3.9943, 14.4505)
  line L558 (3.9943, 14.4505) -> (3.0275, 14.6009)
  line L559 (3.0275, 14.6009) -> (1.9922, 14.7168)
  line L560 (1.9922, 14.7168) -> (0.8898, 14.7914)
  line L561 (0.8898, 14.7914) -> (-0.2784, 14.8179)
  line L562 (-0.2784, 14.8179) -> (-1.4394, 14.7914)
  line L563 (-1.4394, 14.7914) -> (-2.5212, 14.7168)
  line L564 (-2.5212, 14.7168) -> (-3.5244, 14.6009)
  line L565 (-3.5244, 14.6009) -> (-4.4496, 14.4505)
  line L566 (-4.4496, 14.4505) -> (-5.2975, 14.2725)
  line L567 (-5.2975, 14.2725) -> (-6.0685, 14.0739)
  line L568 (-6.0685, 14.0739) -> (-7.3824, 13.6422)
  line L569 (-7.3824, 13.6422) -> (-8.3961, 13.2106)
  line L570 (-8.3961, 13.2106) -> (-9.1144, 12.834)
  line L571 (-9.1144, 12.834) -> (-9.6833, 12.4666)
  line L572 (0, 3.7114) -> (-3.0937, 5.3511)
  line L573 (-3.0937, 5.3511) -> (-1.949, -0.0629)
  line L574 (-1.949, -0.0629) -> (-2.444, -5.1675)
  line L575 (-2.444, -5.1675) -> (0, -6.3432)
  line L576 (0, -6.3432) -> (2.2275, -5.1675)
  line L577 (2.2275, -5.1675) -> (1.8253, -0.0629)
  line L578 (1.8253, -0.0629) -> (2.8772, 5.3511)
  line L579 (2.8772, 5.3511) -> (0, 3.7114)
  line L580 (10.7352, 10.1773) -> (4.455, 5.9698)
  line L581 (4.455, 5.9698) -> (3.4959, 0.5868)
  line L582 (3.4959, 0.5868) -> (9.7761, 0.5868)
  line L583 (9.7761, 0.5868) -> (14.5405, 4.1445)
  line L584 (14.5405, 4.1445) -> (16.1492, 13.3947)
  line L585 (16.1492, 13.3947) -> (11.2302, 12.4666)
  line L586 (11.2302, 12.4666) -> (10.7352, 10.1773)
  line L587 (-2.444, -5.7819) -> (-3.0937, -5.5035)
  line L588 (-3.0937, -5.5035) -> (-3.434, -4.92)
  line L589 (-3.434, -4.92) -> (-5.1046, -5.91)
  line L590 (-5.1046, -5.91) -> (-7.9818, -9.1584)
  line L591 (-7.9818, -9.1584) -> (-9.6833, -9.1584)
  line L592 (-9.6833, -9.1584) -> (-11.1374, -8.6944)
  line L593 (-11.1374, -8.6944) -> (-10.7043, -10.0512)
  line L594 (-10.7043, -10.0512) -> (-9.6833, -10.9528)
  line L595 (-9.6833, -10.9528) -> (-7.9818, -10.9528)
  line L596 (-7.9818, -10.9528) -> (-3.434, -9.9009)
  line L597 (-3.434, -9.9009) -> (0, -8.6944)
  line L598 (0, -8.6944) -> (3.4959, -9.9009)
  line L599 (3.4959, -9.9009) -> (7.889, -10.9528)
  line L600 (7.889, -10.9528) -> (9.7761, -10.9528)
  line L601 (9.7761, -10.9528) -> (10.7352, -10.2412)
  line L602 (10.7352, -10.2412) -> (11.2302, -8.6944)
  line L603 (11.2302, -8.6944) -> (9.7761, -9.1584)
  line L604 (9.7761, -9.1584) -> (7.889, -9.1584)
  line L605 (7.889, -9.1584) -> (4.919, -5.91)
  line L606 (4.919, -5.91) -> (3.2175, -4.92)
  line L607 (3.2175, -4.92) -> (2.8772, -5.5035)
  line L608 (2.8772, -5.5035) -> (2.3512, -5.7819)
  line L609 (2.3512, -5.7819) -> (0, -7.0194)
  line L610 (0, -7.0194) -> (-2.444, -5.7819)
  line L611 (-13.1483, -9.9009) -> (-13.5195, 1.6386)
  line L612 (-13.5195, 1.6386) -> (-10.8899, -0.3104)
  line L613 (-10.8899, -0.3104) -> (-10.8899, -2.7854)
  line L614 (-10.8899, -2.7854) -> (-9.4049, -4.3013)
  line L615 (-9.4049, -4.3013) -> (-9.4049, -8.4778)
  line L616 (-9.4049, -8.4778) -> (-11.1374, -7.9828)
  line L617 (-11.1374, -7.9828) -> (-11.8489, -7.0857)
  line L618 (-11.8489, -7.0857) -> (-11.8489, -8.6944)
  line L619 (-11.8489, -8.6944) -> (-11.1374, -10.5197)
  line L620 (-11.1374, -10.5197) -> (-9.4049, -11.9118)
  line L621 (-9.4049, -11.9118) -> (-9.4049, -13.0565)
  line L622 (-9.4049, -13.0565) -> (-13.1483, -9.9009)
  line L623 (2.2275, -16.0574) -> (-2.444, -16.0574)
  line L624 (-2.444, -16.0574) -> (-1.949, -13.7681)
  line L625 (-1.949, -13.7681) -> (1.8253, -13.7681)
  line L626 (1.8253, -13.7681) -> (2.2275, -16.0574)
  line L627 (3.2175, -3.6516) -> (3.2175, -1.022)
  line L628 (3.2175, -1.022) -> (6.5277, -2.0738)
  line L629 (6.5277, -2.0738) -> (9.4668, -0.6198)
  line L630 (9.4668, -0.6198) -> (9.4668, -2.7854)
  line L631 (9.4668, -2.7854) -> (7.889, -4.3013)
  line L632 (7.889, -4.3013) -> (7.889, -7.7972)
  line L633 (7.889, -7.7972) -> (4.919, -4.5488)
  line L634 (4.919, -4.5488) -> (3.2175, -3.6516)
  line L635 (13.3649, 1.6386) -> (10.7352, -0.3104)
  line L636 (10.7352, -0.3104) -> (10.7352, -2.7854)
  line L637 (10.7352, -2.7854) -> (9.7761, -4.3013)
  line L638 (9.7761, -4.3013) -> (9.7761, -8.4778)
  line L639 (9.7761, -8.4778) -> (11.2302, -7.9828)
  line L640 (11.2302, -7.9828) -> (11.9727, -7.0857)
  line L641 (11.9727, -7.0857) -> (11.9727, -8.6944)
  line L642 (11.9727, -8.6944) -> (11.2302, -10.5197)
  line L643 (11.2302, -10.5197) -> (9.4668, -11.9118)
  line L644 (9.4668, -11.9118) -> (9.4668, -12.84)
  line L645 (9.4668, -12.84) -> (12.9317, -9.9009)
  line L646 (12.9317, -9.9009) -> (13.3649, 1.6386)
  line L647 (5.414, -16.1502) -> (7.889, -13.9537)
  line L648 (7.889, -13.9537) -> (7.889, -12.1284)
  line L649 (7.889, -12.1284) -> (2.6915, -11.1384)
  line L650 (2.6915, -11.1384) -> (-2.444, -11.1384)
  line L651 (-2.444, -11.1384) -> (-7.9818, -12.1284)
  line L652 (-7.9818, -12.1284) -> (-7.9818, -14.2631)
  line L653 (-7.9818, -14.2631) -> (-5.7234, -16.1502)
  line L654 (-5.7234, -16.1502) -> (-4.455, -16.1502)
  line L655 (-4.455, -16.1502) -> (-2.8772, -12.4997)
  line L656 (-2.8772, -12.4997) -> (2.6915, -12.4997)
  line L657 (2.6915, -12.4997) -> (4.2075, -16.1502)
  line L658 (4.2075, -16.1502) -> (5.414, -16.1502)
  line L659 (-5.1046, -4.5488) -> (-7.9818, -7.7972)
  line L660 (-7.9818, -7.7972) -> (-7.9818, -4.0538)
  line L661 (-7.9818, -4.0538) -> (-9.5596, -2.7854)
  line L662 (-9.5596, -2.7854) -> (-9.5596, -0.4651)
  line L663 (-9.5596, -0.4651) -> (-6.6206, -2.0738)
  line L664 (-6.6206, -2.0738) -> (-3.434, -1.022)
  line L665 (-3.434, -1.022) -> (-3.434, -3.6516)
  line L666 (-3.434, -3.6516) -> (-5.1046, -4.5488)
  line L667 (6.0018, 2.8408) -> (6.0018, 1.5414)
  line L668 (6.0018, 1.5414) -> (12.9008, 5.8726)
  line L669 (12.9008, 5.8726) -> (12.9008, 7.2957)
  line L670 (12.9008, 7.2957) -> (6.0018, 2.8408)
  line L671 (6.3421, 5.5633) -> (6.3421, 4.5114)
  line L672 (6.3421, 4.5114) -> (13.5814, 8.9045)
  line L673 (13.5814, 8.9045) -> (13.5814, 10.2966)
  line L674 (13.5814, 10.2966) -> (6.3421, 5.5633)
  line L675 (0.2166, 8.9045) -> (-4.8881, 11.5032)
  line L676 (-4.8881, 11.5032) -> (-4.7822, 11.5665)
  line L677 (-4.7822, 11.5665) -> (-4.5699, 11.632)
  line L678 (-4.5699, 11.632) -> (-4.1804, 11.7081)
  line L679 (-4.1804, 11.7081) -> (-3.5603, 11.7856)
  line L680 (-3.5603, 11.7856) -> (-2.6562, 11.8556)
  line L681 (-2.6562, 11.8556) -> (-1.4151, 11.9088)
  line L682 (-1.4151, 11.9088) -> (0.2166, 11.9363)
  line L683 (0.2166, 11.9363) -> (1.8402, 11.9266)
  line L684 (1.8402, 11.9266) -> (3.0604, 11.8817)
  line L685 (3.0604, 11.8817) -> (3.9346, 11.8128)
  line L686 (3.9346, 11.8128) -> (4.5207, 11.7313)
  line L687 (4.5207, 11.7313) -> (4.8762, 11.6484)
  line L688 (4.8762, 11.6484) -> (5.0587, 11.5752)
  line L689 (5.0587, 11.5752) -> (5.1356, 11.5032)
  line L690 (5.1356, 11.5032) -> (0.2166, 8.9045)
  line L691 (-13.303, 10.2966) -> (-13.303, 8.9045)
  line L692 (-13.303, 8.9045) -> (-5.9709, 4.233)
  line L693 (-5.9709, 4.233) -> (-5.9709, 5.6561)
  line L694 (-5.9709, 5.6561) -> (-13.303, 10.2966)
  line L695 (-12.7461, 7.1101) -> (-12.7461, 5.8726)
  line L696 (-12.7461, 5.8726) -> (-5.7234, 1.3558)
  line L697 (-5.7234, 1.3558) -> (-5.7234, 2.5624)
  line L698 (-5.7234, 2.5624) -> (-12.7461, 7.1101)
  point P0 (0, 0)
  point P1 (0.2166, 8.9045)
  point P2 (0.2166, 11.9363)
  point P3 (15.6233, 3.3711)
  point P4 (0.9589, 16.0796)
  point P5 (-0.2784, 16.0863)
  point P6 (-14.8189, 2.4739)
  point P7 (2.2275, -16.0574)
  point P8 (0, -7.0194)
  point P9 (0, -8.6944)
  point P10 (-1.949, -0.0629)
  point P11 (0, 3.7114)
  point P12 (1.8253, -0.0629)
  point P13 (0, -6.3432)
  point P14 (0, 4.887)
  point P15 (-0.2784, 14.8179)
  point P16 (0.8898, 14.7914)
  point P17 (3.4959, 0.5868)
  point P18 (14.5405, 4.1445)
  point P19 (-3.6196, 0.3702)
  point P20 (-14.8189, 4.1445)
  point P21 (-2.444, -11.1384)
  point P22 (2.6915, -11.1384)
  constraints: 1388 end point
extrude "Wyciągnięcie proste4" cut sketch "Szkic3" against normal blind 1 contours L12 L13 L14 L15 | L16 L17 L18 L19 | L27 L28 L29 L30 | L31 L32 L33 L34 | L74 L73 L72 L71 L70 L69 L68 L67 L66 L65 L64 L63 L62 L61 L60 L59 | L163 L164 L165 L166 L167 L168 L169 L170 L171 L172 L173 L174 L175 L176 L177 L178 L179 L180 L181 L182 L183 L184 L185 L186 L187 L188 L189 L190 L191 L192 L193
extrude "Wyciągnięcie proste5" cut sketch "Szkic3" against normal blind 0.01 contours L11 L10 L9 L8 L7 L6 L5 | L20 L21 L22 L23 L24 L25 L26 | L35 L36 L37 L38 L39 L40 L41 L42 L43 L44 L45 L46 L47 L48 L49 L50 L51 L52 L53 L54 L55 L56 L57 L58 | L75 L76 L77 L78 L79 L80 L81 L82 | L90 L89 L88 L87 L86 L85 L84 L83 | L102 L101 L100 L99 L98 L97 L96 L95 L94 L93 L92 L91 | L103 L104 L105 L106 L107 L108 L109 L110 L111 L112 L113 L114 L115 L116 L117 L118 L119 L120 L121 L122 L123 L124 L125 L126 | L127 L128 L129 L130 L131 L132 L133 L134 L135 L136 L137 L138 | L142 L141 L140 L139 | L150 L149 L148 L147 L146 L145 L144 L143 | L151 L152 L153 L154 L155 L156 L157 L158 L159 L160 L161 L162
ref_plane "Płaszczyzna konstrukcyjna1" through (-40.5, -22, 1) normal (0, -0.5, 0.866) x (1, 0, 0)
sketch "Szkic5" plane through (-40.5, -22, 1) normal (0, -0.5, 0.866) x (1, 0, 0)
  ellipse E0 centre (0, 1.7321) end of major axis (-2, 1.7321) minor radius 1.7321 (-2, 1.7321) -> (0, 0) ccw projected
  line L0 (0, 0) -> (81, 0) projected
  ellipse E1 centre (81, 1.7321) end of major axis (83, 1.7321) minor radius 1.7321 (81, 0) -> (83, 1.7321) ccw projected
  line L1 (83, 1.7321) -> (83, 37.6721) projected
  ellipse E2 centre (81, 37.6721) end of major axis (83, 37.6721) minor radius 1.7321 (83, 37.6721) -> (81, 39.4042) ccw projected
  line L2 (81, 39.4042) -> (0, 39.4042) projected
  ellipse E3 centre (0, 37.6721) end of major axis (-2, 37.6721) minor radius 1.7321 (0, 39.4042) -> (-2, 37.6721) ccw projected
  line L3 (-2, 37.6721) -> (-2, 1.7321) projected
  ellipse E4 centre (80, 35.9401) end of major axis (79, 35.9401) minor radius 0.866 projected
  ellipse E5 centre (1, 35.9401) end of major axis (0, 35.9401) minor radius 0.866 projected
  line L4 (-2, 0) -> (4, 0)
  line L5 (0, 0) -> (81, 0) projected
  line L6 (4, 0) -> (4, 5)
  line L7 (4, 5) -> (19, 5)
  line L8 (19, 5) -> (19, 8)
  line L9 (19, 8) -> (4, 8)
  line L10 (4, 8) -> (4, 5)
  line L11 (19, 14) -> (4, 14)
  line L12 (4, 14) -> (4, 11)
  line L13 (4, 11) -> (19, 11)
  line L14 (19, 11) -> (19, 14)
  line L15 (19, 20) -> (4, 20)
  line L16 (4, 20) -> (4, 17)
  line L17 (4, 17) -> (19, 17)
  line L18 (19, 17) -> (19, 20)
  line L19 (19, 26) -> (4, 26)
  line L20 (4, 26) -> (4, 23)
  line L21 (4, 23) -> (19, 23)
  line L22 (19, 23) -> (19, 26)
  line L23 (19, 32) -> (4, 32)
  line L24 (4, 32) -> (4, 29)
  line L25 (4, 29) -> (19, 29)
  line L26 (19, 29) -> (19, 32)
  line L27 (77, 8) -> (62, 8)
  line L28 (62, 8) -> (62, 5)
  line L29 (62, 5) -> (77, 5)
  line L30 (77, 5) -> (77, 8)
  line L31 (77, 14) -> (62, 14)
  line L32 (62, 14) -> (62, 11)
  line L33 (62, 11) -> (77, 11)
  line L34 (77, 11) -> (77, 14)
  line L35 (77, 20) -> (62, 20)
  line L36 (62, 20) -> (62, 17)
  line L37 (62, 17) -> (77, 17)
  line L38 (77, 17) -> (77, 20)
  line L39 (77, 26) -> (62, 26)
  line L40 (62, 26) -> (62, 23)
  line L41 (62, 23) -> (77, 23)
  line L42 (77, 23) -> (77, 26)
  line L43 (77, 32) -> (62, 32)
  line L44 (62, 32) -> (62, 29)
  line L45 (62, 29) -> (77, 29)
  line L46 (77, 29) -> (77, 32)
  point P0 (40.5, 18.5526)
  dimension "d30" = 6
  dimension "d31" = 5
  dimension "d32" = 90
  dimension "d33" = 15
  dimension "d34" = 3
  dimension "d37" = 6
  dimension "d40" = 58
  constraints: 84 end point, 2 horizontal, 2 parallel, 2 perpendicular, 1 collinear, 1 point on line, 1 vertical, 77 other
  measures "d30" distance of L4.start L4.end
  measures "d31" distance of L4.end L6.end
  measures "d32" angle of L6 L4
  measures "d33" distance of L9.end L8.end
  measures "d34" distance of L8.end L7.end
  measures "d37" distance of L8.end L11.start
  measures "d40" distance of L8.end L27.start
extrude "Wyciągnięcie proste6" cut sketch "Szkic5" against normal through all contours L10 L9 L8 L7 | L14 L13 L12 L11 | L18 L17 L16 L15 | L22 L21 L20 L19 | L26 L25 L24 L23 | L30 L29 L28 L27 | L34 L33 L32 L31 | L38 L37 L36 L35 | L42 L41 L40 L39 | L46 L45 L44 L43
